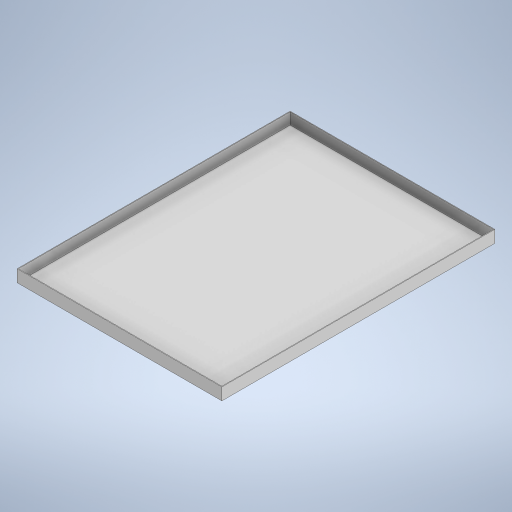
# Autodesk Inventor part: tapa mesa
Saved by Autodesk Inventor 2024 (Build 280153000, 153)
## iProperties
Created: 2023-10-22
Part Number: tapa mesa
Material: Genérico
Document SubType Name: Modeling
Designer: jhonc
Density: 1 g/cm^3
Appearance: Valor por defecto
Author: jhonc
Autodesk Inventor part; units mm, degrees
ref_plane "YZ Plane" through (0, 0, 0) normal (1, 0, 0) x (0, 1, 0)
ref_plane "XZ Plane" through (0, 0, 0) normal (0, 1, 0) x (-1, 0, 0)
ref_plane "XY Plane" through (0, 0, 0) normal (0, 0, 1) x (1, 0, 0)
sketch "Boceto1" plane through (0, 0, 0) normal (0, 1, 0) x (-1, 0, 0)
  line L0 (0, 0) -> (900, 0)
  line L1 (900, 0) -> (900, -1200)
  line L2 (900, -1200) -> (0, -1200)
  line L3 (0, -1200) -> (0, 0)
  dimension "d0" = 900
  dimension "d1" = 1200
  constraints: 8 end point, 2 parallel, 1 horizontal, 1 perpendicular
  measures "d0" distance of L1.end L2.end
  measures "d1" distance of L0.end L1.end
extrude "Extrusión1" add sketch "Boceto1" along normal blind 3
sketch "Boceto2" plane through (0, 3, 0) normal (0, 1, 0) x (1, 0, 0)
  line L0 (0, 1200) -> (-900, 1200) projected
  line L1 (0, 0) -> (-900, 0)
  line L2 (-900, 0) -> (-900, 1200)
  line L3 (-900, 1200) -> (0, 1200)
  line L4 (0, 1200) -> (0, 0)
  line L5 (-897, 1197) -> (-897, 3)
  line L6 (-897, 3) -> (-3, 3)
  line L7 (-3, 3) -> (-3, 1197)
  line L8 (-3, 1197) -> (-897, 1197)
  dimension "d4" = 3
  constraints: 16 end point, 4 parallel, 2 perpendicular, 1 horizontal, 3 other
  measures "d4" distance between parallel lines of L2 L5
extrude "Extrusión2" add sketch "Boceto2" along normal blind 50
